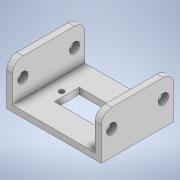
# Autodesk Inventor part: 8_1
Saved by Autodesk Inventor 2021 (Build 250183000, 183)
## iProperties
Created: 2021-04-04
Part Number: 8_1
Material: Genérico
Document SubType Name: Modeling
Designer: diego
Density: 1 g/cm^3
Appearance: Valor por defecto
Author: diego
Autodesk Inventor part; units mm, degrees
ref_plane "YZ Plane" through (0, 0, 0) normal (1, 0, 0) x (0, 1, 0)
ref_plane "XZ Plane" through (0, 0, 0) normal (0, 1, 0) x (-1, 0, 0)
ref_plane "XY Plane" through (0, 0, 0) normal (0, 0, 1) x (1, 0, 0)
sketch "Boceto1" plane through (0, 0, 0) normal (0, 0, 1) x (1, 0, 0)
  line L0 (0, 0) -> (46, 0)
  line L1 (46, 0) -> (46, 21)
  line L2 (46, 21) -> (43, 21)
  line L3 (43, 21) -> (43, 3)
  line L4 (43, 3) -> (3, 3)
  line L5 (3, 3) -> (3, 21)
  line L6 (3, 21) -> (0, 21)
  line L7 (0, 21) -> (0, 0)
  constraints: 16 end point, 5 perpendicular, 2 point on line, 1 horizontal
extrude "Extrusión1" add sketch "Boceto1" against normal blind 35
sketch "Boceto2" plane through (46, 0, 0) normal (1, 0, 0) x (0, 0, -1)
  circle A0 centre (5, 12) radius 2.5
  circle A1 centre (30, 12) radius 2.5
  constraints: 2 centre point
extrude "Extrusión2" cut sketch "Boceto2" against normal blind 60 contours A0
extrude "Extrusión3" cut sketch "Boceto2" against normal blind 60 contours A1
fillet "Empalme1" radius 5 4 edges at (1.5, 21, 0) (1.5, 21, -35) (44.5, 21, 0) (44.5, 21, -35)
sketch "Boceto3" plane through (3, 3, 0) normal (0, 1, 0) x (1, 0, 0)
  line L0 (8.75, 23.5) -> (31.25, 23.5)
  line L1 (31.25, 23.5) -> (31.25, 11.5)
  line L2 (31.25, 11.5) -> (8.75, 11.5)
  line L3 (8.75, 11.5) -> (8.75, 23.5)
  line L4 (8.75, 23.5) -> (8.75, 17.5)
  circle A0 centre (6.25, 17.5) radius 1.25
  line L5 (31.25, 23.5) -> (31.25, 17.5)
  circle A1 centre (33.75, 17.5) radius 1.25
  point P0 (-3, 0)
  point P1 (0, 35)
  constraints: 12 end point, 2 centre point, 2 midpoint, 1 perpendicular
extrude "Extrusión4" cut sketch "Boceto3" against normal blind 60 contours L0 L1 L2 L3
extrude "Extrusión5" cut sketch "Boceto3" against normal blind 60 contours A0 | A1
